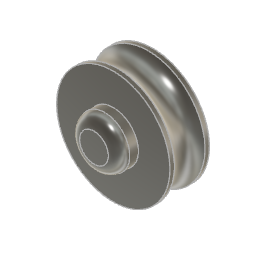
beeboy_wheel (Autodesk Fusion 360 design; units mm, degrees)
Autodesk Fusion 360 part; units mm, degrees
note: some values were not read from the file. Set by a fixed rule: which sketch regions a step uses.
sketch "Sketch1" plane through (0, 0, 0) normal (0, 1, 0) x (1, 0, 0)
  circle A0 centre (0, 0) radius 7.9
  dimension "d1" = 15.8
  constraint coincident A0.centre origin
  measures "d1" diameter of A0
extrude "Extrude1" add sketch "Sketch1" against normal blind 5.5
sketch "Sketch2" plane through (0, -5.5, 0) normal (0, -1, 0) x (1, 0, 0)
  circle A0 centre (0, 0) radius 7.9
  circle A1 centre (0, 0) radius 3.5
  dimension "d4" = 7
  constraint coincident A0.centre A1.centre
  measures "d4" diameter of A1
extrude "Extrude2" add sketch "Sketch2" along normal blind 2.7 contours A1
fillet "Fillet1" radius 1.5 1 edges at (-3.2631, -8.2, -1.2657)
extrude "Extrude3" add 1 faces at (3.1441, 0, -2.759) along direction (0, 1, 0) blind 1.3 draft -73.5
sketch "Sketch3" plane through (0, 1.3, 0) normal (0, 1, 0) x (-1, 0, 0)
  circle A0 centre (0, 0) radius 3.5113
  circle A1 centre (0, 0) radius 1.6
  line L0 (-1.02, 1.2327) -> (-1.02, -1.2327)
  dimension "d11" = 3.2
  dimension "d12" = 1.02
  constraint concentric A0 A1
  constraint coincident A1 L0.start
  constraint coincident A1 L0.end
  constraint vertical L0
  measures "d11" diameter of A1
  measures "d12" distance of A0.centre L0
extrude "Extrude4" cut sketch "Sketch3" against normal blind 9.3 contours A1 L0 picked at (-0.3273, 0.4001)
sketch "Sketch4" plane through (0, 0, 0) normal (1, 0, 0) x (0, 1, 0)
  line L0 (1.3, 0) -> (1.3, -3.5113)
  line L1 (1.3, 3.5113) -> (1.3, 0)
  line L2 (-8.2, 0) -> (-8.2, 2)
  line L3 (-8.2, -2) -> (-8.2, 0)
  line L4 (-5.5, -3.5) -> (-5.5, -7.9)
  line L5 (-5.5, 7.9) -> (-5.5, 3.5)
  line L6 (1.3, 3.5113) -> (0, 7.9)
  line L7 (1.3, -3.5113) -> (0, -7.9)
  arc A0 (-8.2, -2) -> (-6.7, -3.5) centre (-6.7, -2) ccw
  arc A1 (-6.7, 3.5) -> (-8.2, 2) centre (-6.7, 2) ccw
  line L8 (-5.5, 3.5) -> (-6.7, 3.5)
  line L9 (-5.5, -3.5) -> (-6.7, -3.5)
  line L10 (0, 7.9) -> (-5.5, 7.9)
  line L11 (0, -7.9) -> (-5.5, -7.9)
  line L12 (-5.5, 7.9) -> (-5.5, -7.9)
  line L13 (0, -7.9) -> (0, 7.9)
  circle A2 centre (-2.75, 9.2007) radius 2.5
  point P0 (-4.885, 7.9)
  point P1 (-0.615, 7.9)
  dimension "d15" = 0.615
  dimension "d16" = 0.615
  dimension "d17" = 5
  constraint coincident L10 P0
  constraint coincident L10 P1
  constraint coincident P0 A2
  constraint coincident P1 A2
  measures "d15" distance of L5.start P0
  measures "d16" distance of L6.end P1
  measures "d17" diameter of A2
revolve "Revolve1" cut sketch "Sketch4" angle 360 about axis through (0, 1.75, 0) along (0, 1, 0) contours L10 A2 picked at (-2.75, 7.5002)
